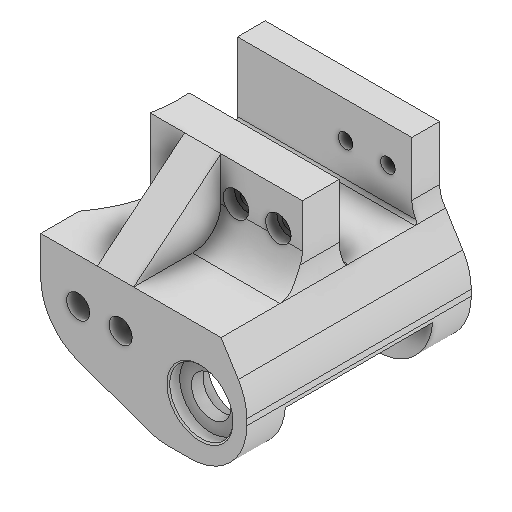
# Autodesk Inventor part: swingarmBaseV4_mirror
Saved by Autodesk Inventor 2025 (Build 290162000, 162)
## iProperties
Created: 2024-10-14
Part Number: swingarmBaseV4_mirror
Material: Generic
Document SubType Name: Modeling
Designer: derm
Density: 1 g/cm^3
Appearance: Default
Author: derm
Autodesk Inventor part; units mm, degrees
ref_plane "YZ Plane" through (0, 0, 0) normal (1, 0, 0) x (0, 1, 0)
ref_plane "XZ Plane" through (0, 0, 0) normal (0, 1, 0) x (-1, 0, 0)
ref_plane "XY Plane" through (0, 0, 0) normal (0, 0, 1) x (1, 0, 0)
sketch "Sketch1" plane through (0, 0, 0) normal (1, 0, 0) x (0, 1, 0)
  line L0 (-12.7635, 12.7635) -> (12.7635, 12.7635)
  line L1 (12.7635, 12.7635) -> (12.7635, -12.7635)
  line L2 (12.7635, -12.7635) -> (-12.7635, -12.7635)
  line L3 (-12.7635, -12.7635) -> (-12.7635, 12.7635)
  line L4 (-12.7635, 12.7635) -> (12.7635, -12.7635) construction
  line L5 (12.7635, 12.7635) -> (-12.7635, -12.7635) construction
  line L6 (19.1135, 19.1135) -> (-19.1135, 19.1135)
  line L7 (-19.1135, 19.1135) -> (-19.1135, -19.1135)
  line L8 (-19.1135, -19.1135) -> (19.1135, -19.1135)
  line L9 (19.1135, -19.1135) -> (19.1135, 19.1135)
  line L10 (12.7635, 19.1135) -> (12.7635, -19.1135)
  line L11 (-19.1135, -5.4793) -> (-46.5737, -5.4793)
  line L12 (-46.5737, -5.4793) -> (-46.5737, -19.1135)
  line L13 (-46.5737, -19.1135) -> (-19.1135, -19.1135)
  line L14 (-19.1135, -19.1135) -> (-19.1135, -5.4793)
  point P0 (0, 0)
  point P1 (12.7635, 12.7635)
  dimension "d1" = 25.527
  dimension "d2" = 6.35
  constraints: 30 end point, 6 parallel, 4 point on line, 3 perpendicular, 2 horizontal, 2 midpoint, 3 other
  measures "d1" distance of L1.end L2.end
  measures "d2" distance between parallel lines of L0 L6
extrude "Extrusion1" add sketch "Sketch1" along normal blind 50.8 contours L13 L12 L11 L7
sketch "Sketch2" plane through (0, -46.5737, -5.4793) normal (0, 0, 1) x (1, 0, 0)
  line L0 (0, 27.4602) -> (0, 0) projected
  line L1 (0, 0) -> (50.8, 0) projected
  line L2 (50.8, 27.4602) -> (50.8, 0) projected
  line L3 (0, 27.4602) -> (50.8, 27.4602) projected
  circle A0 centre (36.2123, 13.7301) radius 7
  point P0 (0, 46.5737)
  dimension "d5" = 14
  constraints: 1 centre point
  measures "d5" diameter of A0
extrude "Extrusion2" cut sketch "Sketch2" against normal through all contours A0
sketch "Sketch7" plane through (0, -46.5737, -5.4793) normal (0, 0, 1) x (1, 0, 0)
  circle A0 centre (36.2123, 13.7301) radius 7 projected
  circle A1 centre (36.2123, 13.7301) radius 11.1875
  point P0 (0, 46.5737)
  dimension "d21" = 22.375
  constraints: 1 centre point, 1 coincident
  measures "d21" diameter of A1
extrude "Extrusion7" cut sketch "Sketch7" against normal blind 4
sketch "Sketch10" plane through (0, -46.5737, -19.1135) normal (0, 0, -1) x (-1, 0, 0)
  circle A0 centre (-36.2123, 13.7301) radius 7 projected
  line L0 (0, 0) -> (0, 27.4602) projected
  line L1 (0, 27.4602) -> (-50.8, 27.4602) projected
  line L2 (-50.8, 0) -> (-50.8, 27.4602) projected
  line L3 (0, 0) -> (-50.8, 0) projected
  circle A1 centre (-36.2123, 13.7301) radius 11
  point P0 (0, 46.5737)
  constraints: 1 centre point, 1 coincident
extrude "Extrusion10" cut sketch "Sketch10" against normal blind 5.5 contours A1
sketch "Sketch11" plane through (0, -46.5737, -5.4793) normal (0, 0, 1) x (1, 0, 0)
  circle A0 centre (36.2123, 13.7301) radius 11.1875 projected
  circle A1 centre (8.2123, 21.7301) radius 2.6
  point P0 (0, 46.5737)
  dimension "d34" = 28
  dimension "d35" = 8
  dimension "d36" = 5.2
  constraints: 1 centre point
  measures "d34" horizontal distance of A0.centre A1.centre
  measures "d35" vertical distance of A0.centre A1.centre
  measures "d36" diameter of A1
extrude "Extrusion11" cut sketch "Sketch11" against normal through all contours A1
sketch "Sketch12" plane through (0, -19.1135, -5.4793) normal (0, 1, 0) x (1, 0, 0)
  line L0 (0, 13.6342) -> (0, 0) projected
  line L1 (0, 0) -> (50.8, 0) projected
  line L2 (50.8, 13.6342) -> (50.8, 0) projected
  line L3 (0, 13.6342) -> (50.8, 13.6342) projected
  point P0 (0, -5.4793)
extrude "Extrusion12" add sketch "Sketch12" along normal blind 10
sketch "Sketch13" plane through (50.8, -46.5737, -19.1135) normal (0, 0, -1) x (-1, 0, 0)
  circle A0 centre (42.5877, 21.7301) radius 2.6 projected
  circle A1 centre (14.5877, 13.7301) radius 11 projected
  line L0 (50.8, 0) -> (50.8, 37.4602) projected
  line L1 (0, 37.4602) -> (50.8, 37.4602) projected
  line L2 (0, 0) -> (0, 37.4602) projected
  line L3 (50.8, 0) -> (0, 0) projected
  line L4 (50.8, 0) -> (50.8, 37.4602) projected
  line L5 (0, 37.4602) -> (50.8, 37.4602)
  line L6 (50.8, 37.4602) -> (50.8, 28.3179)
  line L7 (50.8, 28.3179) -> (14.5877, 28.3179)
  line L8 (0, 28.3179) -> (0, 37.4602)
  arc A2 (14.5877, 28.3179) -> (0, 13.7301) centre (14.5877, 13.7301) ccw
  arc A3 (9.6596, 0) -> (19.5158, 0) centre (14.5877, 13.7301) ccw
  point P0 (50.8, 46.5737)
  constraints: 8 end point, 4 point on circle, 4 point on line, 2 centre point, 2 parallel, 2 tangent, 1 coincident, 1 horizontal, 1 perpendicular
extrude "Extrusion13" add sketch "Sketch13" along normal blind 26 contours L7 A2 L2 L1 L0
mirror "Mirror1" about plane through (25.4, -20.9786, -45.1135) normal (0, 0, -1)
fillet "Fillet5" [suppressed]
sketch "Sketch14" plane through (0, -9.1135, -5.4793) normal (0, 1, 0) x (1, 0, 0)
  line L0 (0, 0) -> (0, 79.2683) projected
  line L1 (0, 0) -> (50.8, 0) projected
  line L2 (50.8, 0) -> (50.8, 79.2683) projected
  line L3 (0, 79.2683) -> (50.8, 79.2683) projected
  circle A0 centre (-6.545, 39.6342) radius 15.197
  point P0 (0, -5.4793)
  constraints: 1 centre point
extrude "Extrusion14" cut sketch "Sketch14" against normal blind 26 contours A0 L0 | L0 A0
fillet "Fillet6" radius 10 2 edges at (0, -13.6847, -31.3981) (0, -13.6847, -58.8289)
sketch "Sketch15" plane through (50.8, -9.1135, -84.7477) normal (0, 0, -1) x (-1, 0, 0)
  line L0 (50.8, -37.4602) -> (0, -37.4602) projected
  line L1 (50.8, -37.4602) -> (50.8, 0) projected
  line L2 (50.8, 0) -> (0, 0) projected
  line L3 (0, -37.4602) -> (0, 0) projected
  circle A0 centre (42.5877, -15.7301) radius 2.6 projected
  circle A1 centre (14.5877, -23.7301) radius 11.1875 projected
  circle A2 centre (-62.5324, 30.9366) radius 78.1359
  point P0 (50.8, 9.1135)
  point P1 (0, -15.9134)
  point P2 (9.2182, 0)
  constraints: 1 centre point
extrude "Extrusion15" cut sketch "Sketch15" against normal through all contours L3 L2 A2 picked at (1.1624, -8.9232)
thicken "Thicken1" operation add thickness 1.5 both sides no extend neighbours no toward (-0.9972038, -0.0747301, 0) faces at (50.7592, -31.7535, -36.4468)
fillet "Fillet7" radius 10 1 edges at (36.2123, -18.2559, -45.1135)
sketch "Sketch16" plane through (0, -9.1135, -5.4793) normal (0, 1, 0) x (1, 0, 0)
  line L0 (41.5818, 0) -> (41.5818, 79.2683) projected
  line L1 (0, 79.2683) -> (41.5818, 79.2683) projected
  line L2 (0, 58.6382) -> (0, 79.2683) projected
  arc A0 (0, 58.6382) -> (3.4337, 51.096) centre (10, 58.6382) ccw projected
  arc A1 (3.4337, 28.1723) -> (3.4337, 51.096) centre (-6.545, 39.6342) ccw projected
  arc A2 (3.4337, 28.1723) -> (0, 20.6301) centre (10, 20.6301) ccw projected
  line L3 (0, 0) -> (0, 20.6301) projected
  line L4 (0, 0) -> (41.5818, 0) projected
  line L5 (0, 0) -> (41.5818, 0)
  line L6 (41.5818, 0) -> (41.5818, 9.8)
  line L7 (41.5818, 9.8) -> (0, 9.8)
  line L8 (0, 9.8) -> (0, 0)
  line L9 (-402.451, 35.28) -> (156.349, 35.28) projected
  line L10 (8.0732, 35.48) -> (41.5818, 35.48)
  line L11 (5.8122, 48.48) -> (41.5818, 48.48)
  line L12 (41.5818, 48.48) -> (36.5818, 48.48)
  line L13 (36.5818, 48.48) -> (36.5818, 79.2683)
  line L14 (36.5818, 79.2683) -> (41.5818, 79.2683)
  line L15 (41.5818, 79.2683) -> (41.5818, 48.48)
  line L16 (5.8122, 48.48) -> (12.8122, 48.48)
  line L17 (12.8122, 48.48) -> (12.8122, 79.2683)
  line L18 (12.8122, 79.2683) -> (5.8122, 79.2683)
  line L19 (5.8122, 79.2683) -> (5.8122, 48.48)
  point P0 (0, -5.4793)
  point P1 (0, 9.8)
  dimension "d54" = 9.8
  dimension "d55" = 0.2
  dimension "d56" = 13
  dimension "d57" = 7
  dimension "d58" = 5
  constraints: 28 end point, 8 parallel, 5 point on line, 3 horizontal, 3 perpendicular, 2 point on circle
  measures "d54" distance between parallel lines of L4 L7
  measures "d55" distance between parallel lines of L9 L10
  measures "d56" distance between parallel lines of L10 L11
  measures "d57" distance between parallel lines of L19 L17
  measures "d58" distance between parallel lines of L0 L13
extrude "Extrusion16" add sketch "Sketch16" along normal blind 25.4 contours L4 L3 L7 L0 | L10 A1 L11 L0 | L19 L1 L17 L11
sketch "Sketch17" plane through (5.8122, -9.1135, -84.7477) normal (-1, 0, 0) x (0, 0, 1)
  line L0 (0, 0) -> (30.7883, 0) projected
  line L1 (0, 0) -> (0, 25.4) projected
  line L2 (30.7883, 25.4) -> (0, 25.4) projected
  line L3 (30.7883, 0) -> (30.7883, 25.4) projected
  line L4 (30.7883, 0) -> (0, 0) projected
  line L5 (30.7883, 0) -> (30.7883, 25.4) projected
  line L6 (0, 0) -> (30.7883, 25.4)
  point P0 (84.7477, 9.1135)
  constraints: 2 end point
extrude "Extrusion17" cut sketch "Sketch17" against normal blind 25.4 contours L1 L2 L6
fillet "Fillet8" radius 10 1 edges at (27.197, -9.1135, -53.9593)
sketch "Sketch18" plane through (-6.545, -18.2559, -45.1135) normal (0, -1, 0) x (1, 0, 0)
  line L0 (37.4895, 26) -> (37.4895, -26) projected
  line L1 (6.545, 26) -> (37.4895, 26) projected
  line L2 (6.545, 26) -> (6.545, 19.004) projected
  arc A0 (6.545, 19.004) -> (9.9788, 11.4619) centre (16.545, 19.004) ccw projected
  arc A1 (9.9788, -11.4619) -> (9.9788, 11.4619) centre (0, 0) ccw projected
  arc A2 (9.9788, -11.4619) -> (6.545, -19.004) centre (16.545, -19.004) ccw projected
  line L3 (6.545, -19.004) -> (6.545, -26) projected
  line L4 (6.545, -26) -> (37.4895, -26) projected
  line L5 (-395.906, 14.7702) -> (-395.906, 19.0981) projected
  line L6 (-395.906, 14.7702) -> (162.894, 14.7702) projected
  line L7 (162.894, 19.0981) -> (162.894, 14.7702) projected
  line L8 (-395.906, 19.0981) -> (162.894, 19.0981) projected
  circle A3 centre (29.9619, 16.9342) radius 2.6
  circle A4 centre (16.545, 16.9342) radius 2.6
  point P0 (6.545, 45.1135)
  dimension "d64" = 5.2
  constraints: 2 centre point
  measures "d64" diameter of A3
extrude "Extrusion18" cut sketch "Sketch18" against normal blind 25.4 contours A3 L6 L8 | L8 A3 | A3 L6 | A4 L8 | L8 A4 L6 | L6 A4
sketch "Sketch19" plane through (-6.545, -18.2559, -45.1135) normal (0, -1, 0) x (1, 0, 0)
  circle A0 centre (16.545, 16.9342) radius 2.6 projected
  circle A1 centre (29.9619, 16.9342) radius 2.6 projected
  circle A2 centre (16.545, 16.9342) radius 4
  circle A3 centre (29.9619, 16.9342) radius 4
  point P0 (6.545, 45.1135)
  dimension "d67" = 8
  dimension "d68" = 8
  constraints: 2 centre point, 2 coincident
  measures "d67" diameter of A3
  measures "d68" diameter of A2
extrude "Extrusion19" cut sketch "Sketch19" against normal blind 5
sketch "Sketch20" plane through (0, -46.5737, -84.7477) normal (0, 0, -1) x (-1, 0, 0)
  circle A0 centre (-8.2123, 21.7301) radius 2.6 projected
  circle A1 centre (-8.2123, 21.7301) radius 4.1
  point P0 (0, 46.5737)
  dimension "d71" = 8.2
  constraints: 1 centre point, 1 coincident
  measures "d71" diameter of A1
extrude "Extrusion20" cut sketch "Sketch20" against normal blind 8 contours A0 | A1
sketch "Sketch21" plane through (0, -46.5737, -5.4793) normal (0, 0, 1) x (1, 0, 0)
  circle A0 centre (8.2123, 21.7301) radius 2.6 projected
  circle A1 centre (8.2123, 21.7301) radius 4.1 projected
  circle A2 centre (8.2123, 21.7301) radius 3.5
  point P0 (0, 46.5737)
  dimension "d74" = 7
  constraints: 1 centre point, 1 coincident
  measures "d74" diameter of A2
extrude "Extrusion21" cut sketch "Sketch21" against normal blind 12 contours A2
sketch "Sketch22" plane through (41.5818, 16.2865, -53.9593) normal (0, 0, -1) x (-1, 0, 0)
  line L0 (444.0328, -10.536) -> (444.0328, -14.864) projected
  line L1 (444.0328, -10.536) -> (-114.7672, -10.536) projected
  line L2 (-114.7672, -14.864) -> (-114.7672, -10.536) projected
  line L3 (444.0328, -14.864) -> (-114.7672, -14.864) projected
  circle A0 centre (8.4648, -12.7) radius 2.6
  circle A1 centre (23.4097, -12.7) radius 2.6
  point P0 (41.5818, -16.2865)
  dimension "d77" = 5.2
  dimension "d78" = 5.2
  constraints: 2 centre point
  measures "d77" diameter of A0
  measures "d78" diameter of A1
extrude "Extrusion22" cut sketch "Sketch22" against normal through all contours A1 L3 L1 | L1 A1 | A1 L3 | A0 L3 L1 | L1 A0 | A0 L3
sketch "Sketch23" plane through (41.5818, 16.2865, -53.9593) normal (0, 0, -1) x (-1, 0, 0)
  circle A0 centre (23.4097, -12.7) radius 2.6 projected
  circle A1 centre (8.4648, -12.7) radius 2.6 projected
  line L0 (28.7696, -15.4) -> (0, -15.4) projected
  line L1 (28.7696, -15.4) -> (28.7696, 0) projected
  line L2 (0, 0) -> (28.7696, 0) projected
  line L3 (0, -15.4) -> (0, 0) projected
  circle A2 centre (8.4648, -12.7) radius 4.5
  circle A3 centre (23.4097, -12.7) radius 4.5
  point P0 (41.5818, -16.2865)
  dimension "d81" = 9
  dimension "d82" = 9
  constraints: 2 centre point, 2 coincident
  measures "d81" diameter of A3
  measures "d82" diameter of A2
extrude "Extrusion23" cut sketch "Sketch23" along normal mid plane 8 contours A0 | A3 L0 | L0 A3 | A2 L0 | L0 A2
ref_plane "Work Plane1" through (41.5818, -9.1135, -28.1193) normal (0, 0, -1) x (-1, 0, 0)
mirror "Mirror2" about plane through (41.5818, -9.1135, -28.1193) normal (0, 0, -1) of "Extrusion23"
fillet "Fillet9" [suppressed]
fillet "Fillet10" radius 5 1 edges at (50.8, -25.0269, -45.1135)
sketch "Sketch24" plane through (0, -46.5737, -84.7477) normal (0, -1, 0) x (1, 0, 0)
  line L0 (0, 79.2683) -> (0, 65.6342) projected
  line L1 (0, 65.6342) -> (50.8, 65.6342) projected
  line L2 (50.8, 79.2683) -> (50.8, 65.6342) projected
  line L3 (0, 79.2683) -> (50.8, 79.2683) projected
  line L4 (0, 0) -> (0, 13.6342) projected
  line L5 (0, 0) -> (50.8, 0) projected
  line L6 (50.8, 0) -> (50.8, 13.6342) projected
  line L7 (0, 13.6342) -> (50.8, 13.6342) projected
  point P0 (0, 84.7477)
extrude "Extrusion24" add sketch "Sketch24" along normal blind 5
sketch "Sketch25" plane through (41.5818, -9.1135, -84.7477) normal (0, 0, -1) x (-1, 0, 0)
  arc A0 (-8.2798, -14.634) -> (-9.2182, -17.5501) centre (-4.2182, -17.5501) ccw projected
  line L0 (-9.2182, -17.5501) -> (-9.2182, -42.4602) projected
  line L1 (41.5818, -42.4602) -> (-9.2182, -42.4602) projected
  line L2 (41.5818, -42.4602) -> (41.5818, 0) projected
  line L3 (41.5818, 0) -> (35.7696, 0) projected
  line L4 (35.7696, 0) -> (28.7696, 0) projected
  line L5 (28.7696, 0) -> (0, 0) projected
  arc A1 (-8.2798, -14.634) -> (0, 0) centre (-71.7506, 30.9366) ccw projected
  circle A2 centre (5.3695, -23.7301) radius 11.1875 projected
  circle A3 centre (33.3695, -15.7301) radius 4.1 projected
  line L6 (5.3695, -42.4602) -> (41.5818, -27.5404)
  point P0 (41.5818, 9.1135)
  constraints: 2 end point, 2 point on line
extrude "Extrusion25" [suppressed]
fillet "Fillet12" [suppressed]
fillet "Fillet13" [suppressed]
chamfer "Chamfer1" distance 0.5 angle 45 2 edges at (25.0248, -32.8436, -5.4793) (25.0248, -32.8436, -84.7477)
chamfer "Chamfer2" distance 3 angle 45 5 edges at (0, -18.2559, -67.6155) (0.8988, -18.2559, -59.974) (8.652, -18.2559, -45.1135) (0.8988, -18.2559, -30.253) (0, -18.2559, -22.6115)
sketch "Sketch26" plane through (30.9444, -18.2559, -71.1135) normal (0, -1, 0) x (1, 0, 0)
  line L0 (-27.9444, 0) -> (-27.9444, 6.996) projected
  line L1 (-27.9444, 0) -> (0, 0) projected
  line L2 (0, 52) -> (0, 0) projected
  line L3 (-27.9444, 52) -> (0, 52) projected
  line L4 (-27.9444, 45.004) -> (-27.9444, 52) projected
  arc A0 (-27.9444, 45.004) -> (-25.5408, 39.7245) centre (-20.9444, 45.004) ccw projected
  arc A1 (-25.5408, 12.2755) -> (-25.5408, 39.7245) centre (-37.4895, 26) ccw projected
  arc A2 (-25.5408, 12.2755) -> (-27.9444, 6.996) centre (-20.9444, 6.996) ccw projected
  circle A3 centre (-7.5276, 42.9342) radius 4 projected
  circle A4 centre (-20.9444, 42.9342) radius 4 projected
  line L5 (-27.9444, 0) -> (-53.6411, 0)
  line L6 (-53.6411, 0) -> (-53.6411, 52)
  line L7 (-53.6411, 52) -> (-27.9444, 52)
  line L8 (-27.9444, 52) -> (-27.9444, 0)
  line L9 (10.6374, 55.8342) -> (-30.9444, 55.8342) projected
  line L10 (10.6374, 17.1542) -> (-18.1322, 17.1542) projected
  line L11 (-30.9444, 6.996) -> (-30.9444, -13.6342) projected
  line L12 (-30.9444, 55.8342) -> (-30.9444, 45.004) projected
  line L13 (-30.9444, 6.996) -> (-30.9444, 0) projected
  line L14 (-30.9444, 0) -> (-30.9444, 52)
  point P0 (-30.9444, 71.1135)
  point P1 (-30.9444, 54.8342)
  constraints: 10 end point, 2 parallel, 2 point on line, 1 horizontal, 1 perpendicular
extrude "Extrusion26" add sketch "Sketch26" against normal up to surface (9.1424 mm away) contours L5 L11 L14 L12 L7 L4 L8 L0 | L8 A0 A1 A2
sketch "Sketch27" plane through (0, -9.1135, -5.4793) normal (0, 1, 0) x (1, 0, 0)
  point P0 (0, -5.4793)
sketch "Sketch28" plane through (0, -9.1135, -5.4793) normal (0, 1, 0) x (1, 0, 0)
  line L0 (12.8122, 48.48) -> (5.8122, 48.48) projected
  arc A0 (8.0732, 35.48) -> (5.8122, 48.48) centre (-6.545, 39.6342) ccw projected
  line L1 (8.0732, 35.48) -> (41.5818, 35.48) projected
  line L2 (41.5818, 35.48) -> (41.5818, 48.48) projected
  line L3 (41.5818, 48.48) -> (12.8122, 48.48) projected
  line L4 (12.8122, 79.2683) -> (12.8122, 48.48) projected
  line L5 (5.8122, 79.2683) -> (12.8122, 79.2683) projected
  line L6 (5.8122, 48.48) -> (5.8122, 79.2683) projected
  line L7 (12.8122, 48.48) -> (5.8122, 48.48) projected
  line L8 (0, 9.8) -> (0, 79.2683) projected
  line L9 (0, 79.2683) -> (5.8122, 79.2683) projected
  line L10 (5.8122, 79.2683) -> (0, 79.2683)
  line L11 (8.0732, 35.48) -> (0, 35.48)
  point P0 (0, -5.4793)
  constraints: 4 end point, 1 horizontal, 1 perpendicular, 1 point on line
extrude "Extrusion27" add sketch "Sketch28" along normal up to surface (25.4 mm away) contours A0 L11 L8 L9 L6
sketch "Sketch29" plane through (5.8122, -9.1135, -84.7477) normal (1, 0, 0) x (0, 0, -1)
  line L0 (-30.7883, 25.4) -> (0, 0) projected
  line L1 (0, 0) -> (0, 25.4) projected
  line L2 (0, 25.4) -> (-30.7883, 25.4) projected
  point P0 (-84.7477, 9.1135)
extrude "Extrusion28" cut sketch "Sketch29" against normal blind 10
sketch "Sketch30" plane through (0, 0, 0) normal (-1, 0, 0) x (0, 0, 1)
  line L0 (-53.9593, 16.2865) -> (-84.7477, -9.1135) projected
  line L1 (-84.7477, -51.5737) -> (-84.7477, -9.1135) projected
  line L2 (-71.1135, -51.5737) -> (-84.7477, -51.5737) projected
  line L3 (-71.1135, -51.5737) -> (-71.1135, -18.2559) projected
  line L4 (-19.1135, -18.2559) -> (-71.1135, -18.2559) projected
  line L5 (-19.1135, -18.2559) -> (-19.1135, -51.5737) projected
  line L6 (-5.4793, -51.5737) -> (-19.1135, -51.5737) projected
  line L7 (-5.4793, -51.5737) -> (-5.4793, 16.2865) projected
  line L8 (-15.2793, 16.2865) -> (-5.4793, 16.2865) projected
  line L9 (-15.2793, -9.1135) -> (-15.2793, 16.2865) projected
  line L10 (-15.2793, -9.1135) -> (-40.9593, -9.1135) projected
  line L11 (-40.9593, -9.1135) -> (-40.9593, 16.2865) projected
  line L12 (-40.9593, 16.2865) -> (-53.9593, 16.2865) projected
  line L13 (-40.9593, -9.1135) -> (-63.9593, -9.1135) projected
  line L14 (-84.7477, -9.1135) -> (-63.9593, -9.1135) projected
  line L15 (-40.9593, -9.1135) -> (-84.7477, -9.1135)
  line L16 (-84.7477, -9.1135) -> (-5.4793, -9.1135)
  point P0 (0, 0)
  constraints: 4 end point, 2 point on line, 1 collinear
extrude "Extrusion29" add sketch "Sketch30" along normal blind 20 contours L14 L13 L10 L16 L7 L6 L5 L4 L3 L2 L1
pattern_linear "Rectangular Pattern1" count 2 spacing 15 along (-1, 0, 0) of "Extrusion20", "Extrusion21", "Extrusion11"
sketch "Sketch31" plane through (-6.7877, -24.8436, -17.4793) normal (0, 0, 1) x (1, 0, 0)
  circle A0 centre (0, 0) radius 2.6 projected
  point P0 (6.7877, 24.8436)
extrude "Extrusion30" cut sketch "Sketch31" against normal through all
sketch "Sketch32" plane through (0, -9.1135, -5.4793) normal (0, 1, 0) x (1, 0, 0)
  line L0 (-20, 65.6342) -> (30.9444, 65.6342) projected
  line L1 (30.9444, 13.6342) -> (30.9444, 65.6342) projected
  line L2 (-20, 13.6342) -> (30.9444, 13.6342) projected
  line L3 (-20, 65.6342) -> (-20, 13.6342) projected
  circle A0 centre (23.4168, 22.7) radius 4 projected
  circle A1 centre (10, 22.7) radius 4 projected
  line L4 (-20, 65.6342) -> (-20, 13.6342) projected
  arc A2 (-20, 13.6342) -> (-20, 65.6342) centre (-54.1681, 39.6342) ccw
  point P0 (0, -5.4793)
  constraints: 2 point on circle, 1 centre point
extrude "Extrusion31" cut sketch "Sketch32" against normal blind 10 contours A2 L3
sketch "Sketch33" plane through (0, -9.1135, -5.4793) normal (0, 1, 0) x (1, 0, 0)
  line L0 (0, 9.8) -> (0, 0) projected
  line L1 (0, 0) -> (41.5818, 0) projected
  line L2 (41.5818, 0) -> (41.5818, 9.8) projected
  line L3 (41.5818, 9.8) -> (0, 9.8) projected
  line L4 (12.8122, 48.48) -> (0, 48.48) projected
  line L5 (0, 35.48) -> (0, 48.48) projected
  line L6 (41.5818, 35.48) -> (0, 35.48) projected
  line L7 (41.5818, 35.48) -> (41.5818, 48.48) projected
  line L8 (41.5818, 48.48) -> (12.8122, 48.48) projected
  arc A0 (-20, 13.6342) -> (-20, 65.6342) centre (-54.1681, 39.6342) ccw projected
  line L9 (-20, 0) -> (-20, 13.6342) projected
  line L10 (0, 0) -> (-20, 0) projected
  line L11 (0, 9.8) -> (0, 0) projected
  line L12 (0, 9.8) -> (41.5818, 9.8) projected
  line L13 (41.5818, 9.8) -> (41.5818, 35.48) projected
  line L14 (41.5818, 35.48) -> (0, 35.48) projected
  line L15 (0, 79.2683) -> (0, 35.48) projected
  line L16 (0, 79.2683) -> (-20, 79.2683) projected
  line L17 (-20, 65.6342) -> (-20, 79.2683) projected
  circle A1 centre (10, 22.7) radius 2.6 projected
  circle A2 centre (23.4168, 22.7) radius 2.6 projected
  line L18 (0, 9.8) -> (-20, 9.8)
  line L19 (0, 48.48) -> (-12.1537, 48.48)
  line L20 (0, 35.48) -> (-11.434, 35.48)
  point P0 (0, -5.4793)
  constraints: 6 end point, 2 point on circle, 2 point on line, 1 parallel, 1 perpendicular
extrude "Extrusion32" add sketch "Sketch33" along normal up to surface (25.4 mm away) contours L0 L10 L9 L18 | L20 A0 L19 L5
fillet "Fillet14" radius 1 2 edges at (10.7909, -9.1135, -15.2793) (15.0739, -9.1135, -40.9593)
sketch "Sketch34" plane through (41.5818, -9.1135, -84.7477) normal (0, 0, -1) x (-1, 0, 0)
  circle A0 centre (48.3695, -15.7301) radius 4.1 projected
  line L0 (41.5818, 0) -> (28.7696, 0) projected
  line L1 (28.7696, 0) -> (0, 0) projected
  arc A1 (-8.2798, -14.634) -> (0, 0) centre (-71.7506, 30.9366) ccw projected
  arc A2 (-8.2798, -14.634) -> (-9.2182, -17.5501) centre (-4.2182, -17.5501) ccw projected
  line L2 (-9.2182, -17.5501) -> (-9.2182, -42.4602) projected
  line L3 (-9.2182, -42.4602) -> (61.5818, -42.4602) projected
  line L4 (61.5818, 0) -> (61.5818, -42.4602) projected
  line L5 (41.5818, 0) -> (61.5818, 0) projected
  circle A3 centre (33.3695, -15.7301) radius 4.1 projected
  circle A4 centre (5.3695, -23.7301) radius 11.6875 projected
  line L6 (0, 10) -> (0, 0) projected
  line L7 (0, 0) -> (-2.106, 0)
  line L8 (-2.106, 0) -> (-11.1734, -14.634)
  line L9 (-11.1734, -14.634) -> (-11.1734, -42.4602)
  line L10 (-11.1734, -42.4602) -> (-9.2182, -42.4602)
  point P0 (41.5818, 9.1135)
  constraints: 8 end point, 2 perpendicular, 1 horizontal
extrude "Extrusion33" add sketch "Sketch34" against normal up to surface (79.2683 mm away) contours A1 A2 L2 L10 L9 L8 L7
sketch "Sketch35" plane through (50.8, -51.5737, -71.1135) normal (-1, 0, 0) x (0, 0, 1)
  line L0 (0, 0) -> (0, 18.7301) projected
  line L1 (0, 0) -> (52, 0) projected
  line L2 (52, 18.7301) -> (52, 0) projected
  line L3 (52, 18.7301) -> (0, 18.7301) projected
  point P0 (71.1135, 51.5737)
extrude "Extrusion34" cut sketch "Sketch35" against normal blind 10
sketch "Sketch36" plane through (12.8122, -9.1135, -84.7477) normal (0, 0, -1) x (-1, 0, 0)
  circle A0 centre (19.5999, -15.7301) radius 4.1 projected
  line L0 (12.8122, 0) -> (0, 0) projected
  line L1 (0, 0) -> (-30.8757, 0) projected
  line L2 (-30.8757, 0) -> (-39.943, -14.634) projected
  line L3 (-39.943, -14.634) -> (-39.943, -42.4602) projected
  line L4 (-39.943, -42.4602) -> (32.8122, -42.4602) projected
  line L5 (32.8122, 0) -> (32.8122, -42.4602) projected
  line L6 (12.8122, 0) -> (32.8122, 0) projected
  circle A1 centre (4.5999, -15.7301) radius 4.1 projected
  circle A2 centre (-23.4001, -23.7301) radius 11.6875 projected
  line L7 (32.8122, -27.7337) -> (-8.6304, -42.4602)
  line L8 (-39.943, -42.4602) -> (32.8122, -42.4602) projected
  point P0 (12.8122, 9.1135)
  point P1 (-8.6304, -42.4602)
  constraints: 2 end point, 2 point on line
extrude "Extrusion35" cut sketch "Sketch36" against normal through all contours L5 L4 L7
fillet "Fillet15" radius 20 7 edges at (52.7552, -51.5737, -77.9306) (21.4426, -51.5737, -77.9306) (-20, -36.8472, -77.9306) (21.4426, -51.5737, -12.2964) (-20, -36.8472, -12.2964) (52.7552, -51.5737, -12.2964) (52.7552, -23.7475, -45.1135)
sketch "Sketch37" plane through (-20, -18.2559, -71.1135) normal (0, 0, 1) x (1, 0, 0)
  circle A0 centre (28.2123, -6.5877) radius 2.6 projected
  circle A1 centre (56.2123, -14.5877) radius 11 projected
  circle A2 centre (13.2123, -6.5877) radius 2.6 projected
  arc A3 (0, -4.4731) -> (13.3033, -23.3187) centre (20, -4.4731) ccw projected
  line L0 (13.3033, -23.3187) -> (38.1938, -32.1634) projected
  arc A4 (38.1938, -32.1634) -> (44.8905, -33.3179) centre (44.8905, -13.3179) ccw projected
  line L1 (52.7552, -33.3179) -> (44.8905, -33.3179) projected
  arc A5 (52.7552, -33.3179) -> (72.7148, -14.5877) centre (52.7552, -13.3179) ccw projected
  line L2 (69.3, -14.5877) -> (72.7148, -14.5877) projected
  arc A6 (69.3, -14.5877) -> (56.2123, -1.5) centre (56.2123, -14.5877) ccw projected
  arc A7 (56.2123, -1.5) -> (50.9444, 0) centre (50.9444, -10) ccw projected
  line L3 (0, 0) -> (50.9444, 0) projected
  line L4 (0, -4.4731) -> (0, 0) projected
  line L5 (0.5636, -9.1877) -> (6.223, -9.1877)
  line L6 (6.223, -9.1877) -> (23.2037, -13.3179)
  line L7 (23.2037, -13.3179) -> (25.4722, -27.6428)
  point P0 (20, 18.2559)
  constraints: 6 end point, 1 horizontal, 1 point on circle, 1 point on line
extrude "Extrusion36" cut sketch "Sketch37" against normal blind 6 contours L5 L6 L7 L0 A3
fillet "Fillet16" radius 5 2 edges at (-13.777, -27.4436, -74.1135) (3.2037, -31.5737, -74.1135)
fillet "Fillet18" radius 10 1 edges at (5.4722, -45.8987, -74.1135)
fillet "Fillet19" radius 10 2 edges at (41.5818, -9.1135, -10.8793) (41.5818, -9.1135, -51.9593)
mirror "Mirror3" about plane through (0, -19.1135, -5.4793) normal (0, 0, 1) remove original yes
body "Solid1"
